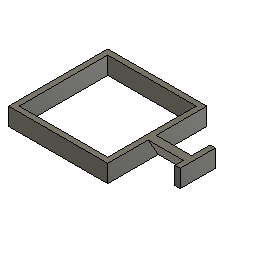
IPA Tweezer Mount v4 (Autodesk Fusion 360 design; units mm, degrees)
Autodesk Fusion 360 part; units mm, degrees
sketch "Base Mount Sketch" plane through (0, 0, 0) normal (0, 1, 0) x (1, 0, 0) in component "Mount"
  line L0 (0, 0) -> (50.2, 0)
  line L1 (50.2, 0) -> (50.2, 50.2)
  line L2 (50.2, 50.2) -> (0, 50.2)
  line L3 (0, 50.2) -> (0, 0)
  line L4 (73.2, 35.1) -> (76.2, 35.1)
  line L5 (76.2, 35.1) -> (76.2, 15.1)
  line L6 (76.2, 15.1) -> (73.2, 15.1)
  line L7 (73.2, 15.1) -> (73.2, 35.1)
  line L8 (0, 25.1) -> (53.2, 25.1) construction
  line L9 (73.2, 23.6) -> (53.2, 23.6)
  line L10 (53.2, 23.6) -> (53.2, -3)
  line L11 (53.2, -3) -> (-3, -3)
  line L12 (-3, -3) -> (-3, 53.2)
  line L13 (-3, 53.2) -> (53.2, 53.2)
  line L14 (53.2, 53.2) -> (53.2, 26.6)
  line L15 (53.2, 26.6) -> (73.2, 26.6)
  line L16 (53.2, 26.6) -> (53.2, 23.6)
  line L17 (53.2, 25.1) -> (73.2, 25.1) construction
  dimension "d1" = 50.2
  dimension "d2" = 50.2
  dimension "d5" = 3
  dimension "d6" = 20
  dimension "d8" = 3
  dimension "d9" = 3
  dimension "d10" = 3
  dimension "d11" = 3
  dimension "d12" = 3
  dimension "d13" = 20
  constraint horizontal L0
  constraint vertical L1
  constraint horizontal L2
  constraint vertical L3
  constraint coincident L0.start L3.end
  constraint horizontal L4
  constraint vertical L5
  constraint horizontal L6
  constraint vertical L7
  constraint midpoint L3 L8.start
  constraint midpoint L7 L17.end
  constraint horizontal L8
  constraint coincident L7 L9.start
  constraint perpendicular L7 L9
  constraint perpendicular L9 L10
  constraint perpendicular L7 L13
  constraint coincident L7 L15.end
  constraint perpendicular L7 L15
  constraint vertical L12
  constraint vertical L14
  constraint horizontal L11
  constraint collinear L10 L14
  constraint coincident L16 L8.end
  constraint horizontal L17
  constraint midpoint L16 L8.end
  measures "d1" distance of L0.start L0.end
  measures "d2" distance of L0.start L2.end
  measures "d5" distance of L5 L7
  measures "d6" distance of L4 L6
  measures "d8" distance of L3 L12
  measures "d9" distance of L2 L13
  measures "d10" distance of L0 L11
  measures "d11" distance of L1 L10
  measures "d12" distance of L9 L15
  measures "d13" distance of L7 L14
extrude "Extrude1" add sketch "Base Mount Sketch" along normal blind 10 contours L10 L11 L12 L13 L14 L16 in component "Mount"
sketch "Tweezer Mount Tilt sketch" plane through (53.2, 0, 0) normal (1, 0, 0) x (0, 0, -1) in component "Mount"
  line L0 (-3, 0) -> (53.2, 0)
  line L1 (53.2, 0) -> (53.2, 10)
  line L2 (53.2, 10) -> (-3, 10)
  line L3 (-3, 10) -> (-3, 0)
  line L4 (25.1, 0) -> (25.1, 10) construction
  line L5 (30.2962, 0) -> (24.5226, 10)
  line L6 (25.6774, 0) -> (19.9038, 10)
  line L7 (25.1, 5) -> (30.2962, 0) construction
  line L8 (25.6774, 0) -> (24.5226, 10) construction
  line L9 (19.9038, 10) -> (25.1, 5) construction
  dimension "d25" = 4
  dimension "d32" = 60
  constraint midpoint L0 L4.start
  constraint midpoint L2 L4.end
  constraint coincident L0 L5.start
  constraint coincident L2 L5.end
  constraint coincident L0 L6.start
  constraint coincident L2 L6.end
  constraint parallel L5 L6
  constraint coincident L8 L7.start
  constraint midpoint L4 L7.start
  measures "d25" distance of L5 L6
  measures "d32" angle of L0 L6
extrude "Extrude2" add sketch "Tweezer Mount Tilt sketch" along normal blind 20 contours L0 L2 L5 L6 in component "Mount"
extrude "Extrude3" add sketch "Base Mount Sketch" along normal blind 10 contours L4 L5 L6 L7 in component "Mount"
component "Mount" placed x (1, 0, 0) y (0, 1, 0) z (0, 0, 1) at (0, 0, 0)
equation "d1 = IPA_container_size + fitting_clearance"
equation "d2 = IPA_container_size + fitting_clearance"
equation "nominal_thickness = 3 mm"
equation "IPA_container_size = 50 mm"
equation "d5 = nominal_thickness"
equation "d6 = stopend_width"
equation "d8 = nominal_thickness"
equation "d9 = nominal_thickness"
equation "d10 = nominal_thickness"
equation "d11 = nominal_thickness"
equation "d12 = nominal_thickness"
equation "d13 = tweezer_mount_width"
equation "tweezer_mount_width = 20 mm"
equation "stopend_width = 20 mm"
equation "fitting_clearance = 0.2 mm"
equation "attachment_height = 10 mm"
equation "d18 = attachment_height"
equation "d25 = tweezer_mount_thickness"
equation "tweezer_mount_thickness = nominal_thickness + 1 mm"
equation "d27 = tweezer_mount_width"
equation "d29 = attachment_height"
equation "tweezer_mount_tilt_angle = 60 deg"
equation "d32 = tweezer_mount_tilt_angle"
named bodies: "Attachment"
